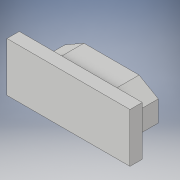
# Autodesk Inventor part: ChargeCover
Saved by Autodesk Inventor 2019 (Build 230136000, 136)
## iProperties
Created: 2021-04-26
Part Number: ChargeCover
Material: Všeobecné
Document SubType Name: Modeling
Designer: miko flosso
Density: 1 g/cm^3
Appearance: Výchozí
Author: miko flosso
Autodesk Inventor part; units mm, degrees
ref_plane "YZ Plane" through (0, 0, 0) normal (1, 0, 0) x (0, 1, 0)
ref_plane "XZ Plane" through (0, 0, 0) normal (0, 1, 0) x (-1, 0, 0)
ref_plane "XY Plane" through (0, 0, 0) normal (0, 0, 1) x (1, 0, 0)
sketch "Náčrt1" plane through (0, 0, 0) normal (0, 0, 1) x (1, 0, 0)
  line L0 (0, 0) -> (7.6, 0)
  line L1 (7.6, 0) -> (7.6, 2.6)
  line L2 (7.6, 2.6) -> (0, 2.6)
  line L3 (0, 2.6) -> (0, 0)
  dimension "d0" = 7.6
  dimension "d1" = 2.6
  constraints: 8 end point, 2 parallel, 1 horizontal, 1 perpendicular
  measures "d0" distance of L2.end L1.end
  measures "d1" distance of L1.end L0.end
extrude "Vysunutí1" add sketch "Náčrt1" along normal blind 2.5
chamfer "Zkosení1" distance 0.9 angle 60 1 edges at (0, 2.6, 1.25) measured on face at (0, 1.7333, 0.8333)
chamfer "Zkosení2" distance 0.9 angle 60 1 edges at (7.6, 2.6, 1.25) measured on face at (7.6, 0.8667, 0.8333)
sketch "Náčrt2" plane through (0, 0, 2.5) normal (0, 0, 1) x (1, 0, 0)
  line L0 (-1.2, -0.7) -> (8.8, -0.7)
  line L1 (8.8, -0.7) -> (8.8, 3.3)
  line L2 (8.8, 3.3) -> (-1.2, 3.3)
  line L3 (-1.2, 3.3) -> (-1.2, -0.7)
  line L4 (-1.2, -0.7) -> (8.8, 3.3) construction
  line L5 (8.8, -0.7) -> (-1.2, 3.3) construction
  line L6 (0, 0) -> (7.6, 0) projected
  point P0 (3.8, 1.3)
  dimension "d10" = 10
  dimension "d11" = 4
  dimension "d12" = 1.3
  constraints: 12 end point, 2 midpoint, 2 parallel, 1 horizontal, 1 perpendicular
  measures "d10" distance of L2.end L1.end
  measures "d11" distance of L1.end L0.end
  measures "d12" distance from line of L6 point (3.8, 1.3)
extrude "Vysunutí2" add sketch "Náčrt2" along normal blind 1
